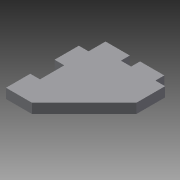
# Autodesk Inventor part: FDM20-BasePrincipal-PortaMotorY-Lateral-01
Saved by Autodesk Inventor 2015 (Build 190159000, 159)
## iProperties
Created: 2016-02-23
Part Number: FDM20-BasePrincipal-PortaMotorY-Lateral-01
Material: Generic
Document SubType Name: Modeling
Designer: Proyectil
Density: 1 g/cm^3
Appearance: Default
Author: Proyectil
Autodesk Inventor part; units mm, degrees
ref_plane "YZ Plane" through (0, 0, 0) normal (1, 0, 0) x (0, 1, 0)
ref_plane "XZ Plane" through (0, 0, 0) normal (0, 1, 0) x (-1, 0, 0)
ref_plane "XY Plane" through (0, 0, 0) normal (0, 0, 1) x (1, 0, 0)
sketch "Sketch1" plane through (0, 0, 0) normal (0, 0, 1) x (1, 0, 0)
  line L0 (15, -5.5) -> (0, -5.5) projected
  line L1 (15, 0) -> (15, -5.5) projected
  line L2 (0, 0) -> (15, 0) projected
  line L3 (0, 0) -> (0, -5.5) projected
  line L4 (-6.3, -5.5) -> (-21.3, -5.5) projected
  line L5 (-6.3, 0) -> (-6.3, -5.5) projected
  line L6 (-21.3, 0) -> (-6.3, 0) projected
  line L7 (-21.3, 0) -> (-21.3, -5.5) projected
  line L8 (-27.3, 0) -> (-27.3, -5.5) projected
  line L9 (21, 0) -> (21, -5.5) projected
  line L10 (-21.3, -5.5) -> (-21.3, -55.5)
  line L11 (-21.3, -55.5) -> (-11.3, -55.5)
  line L12 (-11.3, -55.5) -> (21, -23.2)
  line L13 (21, -23.2) -> (21, -5.5)
  line L14 (21, 0) -> (15, 0)
  line L15 (0, 0) -> (-6.3, 0)
  line L16 (-21.3, -55.5) -> (-27.3, -55.5)
  line L17 (-27.3, -55.5) -> (-27.3, -40.5)
  line L18 (-27.3, -40.5) -> (-21.3, -40.5)
  line L19 (-21.3, -40.5) -> (-21.3, -55.5)
  line L20 (-21.3, -25.5) -> (-27.3, -25.5)
  line L21 (-27.3, -25.5) -> (-27.3, -10.5)
  line L22 (-27.3, -10.5) -> (-21.3, -10.5)
  line L23 (-21.3, -10.5) -> (-21.3, -25.5)
  line L24 (-6.3, -5.5) -> (0, -5.5)
  line L25 (15, -5.5) -> (21, -5.5)
  dimension "d0" = 50
  dimension "d1" = 10
  dimension "d2" = 135
  dimension "d3" = 6
  dimension "d4" = 15
  dimension "d5" = 15
  dimension "d6" = 15
  constraints: 32 end point, 5 parallel, 4 horizontal, 4 perpendicular, 2 point on line, 1 collinear, 1 vertical
  measures "d0" distance of L4.end L10.end
  measures "d1" distance of L10.end L11.end
  measures "d2" angle of L12 L11
  measures "d3" distance of L17.end L18.end
  measures "d4" distance of L16.end L17.end
  measures "d5" distance of L20.end L21.end
  measures "d6" distance between parallel lines of L20 L18
extrude "Extrusion1" add sketch "Sketch1" along normal blind 6 contours L25 L13 L12 L11 L10 L4 L24 L0 | L0 L3 L2 L1 | L4 L7 L6 L5 | L10 L20 L21 L22 | L16 L17 L18 L10
sketch "Sketch2" plane through (0, 0, 6) normal (0, 0, 1) x (1, 0, 0)
  line L0 (0, -5.5) -> (-6.3, -5.5) construction
  line L1 (-3.15, -5.5) -> (-3.15, -15.5) construction
  line L2 (-4.9, -5.5) -> (-4.9, -10.5)
  line L3 (-4.9, -10.5) -> (-5.9, -10.5)
  line L4 (-5.9, -10.5) -> (-5.9, -12.5)
  line L5 (-5.9, -12.5) -> (-4.9, -12.5)
  line L6 (-4.9, -12.5) -> (-4.9, -15.5)
  line L7 (-4.9, -15.5) -> (-1.4, -15.5)
  line L8 (-1.4, -15.5) -> (-1.4, -12.5)
  line L9 (-1.4, -12.5) -> (-0.4, -12.5)
  line L10 (-0.4, -12.5) -> (-0.4, -10.5)
  line L11 (-0.4, -10.5) -> (-1.4, -10.5)
  line L12 (-1.4, -10.5) -> (-1.4, -5.5)
  line L13 (-1.4, -5.5) -> (-4.9, -5.5)
  line L14 (-21.3, -25.5) -> (-21.3, -40.5) construction
  line L15 (-21.3, -33) -> (-11.3, -33) construction
  line L16 (-21.3, -31.25) -> (-16.3, -31.25)
  line L17 (-16.3, -31.25) -> (-16.3, -30.25)
  line L18 (-16.3, -30.25) -> (-14.3, -30.25)
  line L19 (-14.3, -30.25) -> (-14.3, -31.25)
  line L20 (-14.3, -31.25) -> (-11.3, -31.25)
  line L21 (-11.3, -31.25) -> (-11.3, -34.75)
  line L22 (-11.3, -34.75) -> (-14.3, -34.75)
  line L23 (-14.3, -34.75) -> (-14.3, -35.75)
  line L24 (-14.3, -35.75) -> (-16.3, -35.75)
  line L25 (-16.3, -35.75) -> (-16.3, -34.75)
  line L26 (-16.3, -34.75) -> (-21.3, -34.75)
  line L27 (-21.3, -31.25) -> (-21.3, -34.75)
  point P0 (0, 0)
  dimension "d9" = 10
  dimension "d10" = 5
  dimension "d11" = 2
  dimension "d12" = 3
  dimension "d13" = 3.5
  dimension "d14" = 1.75
  dimension "d15" = 5.5
  dimension "d16" = 2.75
  dimension "d19" = 10
  dimension "d20" = 5
  dimension "d21" = 2
  dimension "d22" = 3
  dimension "d23" = 3.5
  dimension "d24" = 1.75
  dimension "d25" = 2
  dimension "d26" = 5.5
  dimension "d27" = 2.75
  constraints: 52 end point, 15 perpendicular, 12 point on line, 3 collinear, 3 horizontal, 3 vertical, 2 midpoint
  measures "d9" distance of L1.start L1.end
  measures "d10" distance of L2.start L2.end
  measures "d11" distance of L3.end L4.end
  measures "d12" distance of L5.end L6.end
  measures "d13" distance of L6.end L7.end
  measures "d14" distance between parallel lines of L1 L2
  measures "d15" distance between parallel lines of L10 L4
  measures "d16" distance between parallel lines of L1 L10
  measures "d19" distance of L15.start L15.end
  measures "d20" distance of L16.start L16.end
  measures "d21" distance of L17.end L18.end
  measures "d22" distance of L19.end L20.end
  measures "d23" distance of L20.end L21.end
  measures "d24" distance between parallel lines of L15 L16
  measures "d25" distance of L23.end L24.end
  measures "d26" distance between parallel lines of L24 L18
  measures "d27" distance between parallel lines of L15 L18
extrude "Extrusion2" cut sketch "Sketch2" against normal up to next
equation "\"d16\" = 0.5 * d15"
equation "\"d24\" = 0.5 * d23"
equation "\"d27\" = 0.5 * d26"
body "Solid1"
